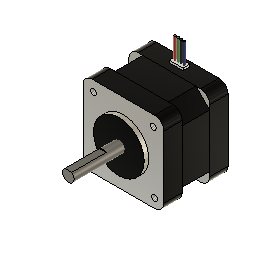
Nema14-Generic (Autodesk Fusion 360 design; units mm, degrees)
Autodesk Fusion 360 part; units mm, degrees
sketch "Profile" plane through (0, 0, 0) normal (0, 1, 0) x (1, 0, 0)
  line L0 (17.6, -17.6) -> (-17.6, -17.6)
  line L1 (-17.6, -17.6) -> (-17.6, 17.6)
  line L2 (-17.6, 17.6) -> (17.6, 17.6)
  line L3 (17.6, 17.6) -> (17.6, -17.6)
  line L4 (17.6, -17.6) -> (-17.6, 17.6) construction
  line L5 (-17.6, -17.6) -> (17.6, 17.6) construction
  circle A0 centre (0, 0) radius 11
  circle A1 centre (0, 0) radius 2.5
  line L6 (-1.5, -2) -> (1.5, -2)
  circle A2 centre (0, 0) radius 18.3848 construction
  line L7 (-11.6, -17.6) -> (-17.6, -11.6)
  line L8 (0, 0) -> (0, -17.6) construction
  line L9 (0, 0) -> (-17.6, 0) construction
  line L10 (11.6, -17.6) -> (17.6, -11.6)
  line L11 (-11.6, 17.6) -> (-17.6, 11.6)
  line L12 (11.6, 17.6) -> (17.6, 11.6)
  point P0 (0, 2.5)
  point P1 (-13, -13)
  point P2 (13, -13)
  point P3 (13, 13)
  point P4 (-13, 13)
  dimension "d1" = 35.2
  dimension "d2" = 22
  dimension "d3" = 5
  dimension "d5" = 4.5
  dimension "d8" = 26
  dimension "d18" = 6
  constraint horizontal L0
  constraint perpendicular L0 L1
  constraint parallel L0 L2
  constraint parallel L1 L3
  constraint coincident L4 A0.centre
  constraint coincident L5 A0.centre
  constraint coincident A0.centre A1.centre
  constraint equal L0 L3
  constraint coincident A1 L6.start
  constraint coincident A1 L6.end
  constraint horizontal L6
  constraint coincident A1 P0
  constraint vertical A0.centre P0
  constraint coincident A2 P1
  constraint coincident L5 P1
  constraint coincident A2 P2
  constraint coincident L4 P2
  constraint coincident A2 P3
  constraint coincident L5 P3
  constraint coincident A2 P4
  constraint coincident L4 P4
  constraint coincident L0 L7.start
  constraint coincident L1 L7.end
  constraint perpendicular L5 L7
  constraint midpoint L0 L8.end
  constraint midpoint L1 L9.end
  constraint symmetric L7.start L8 L10.start
  constraint symmetric L7.end L8 L10.end
  constraint symmetric L7.start L9 L11.start
  constraint symmetric L7.end L9 L11.end
  constraint symmetric L9 L10.start L12.start
  constraint symmetric L9 L10.end L12.end
  measures "d1" distance of L0.start L0.end
  measures "d2" diameter of A0
  measures "d3" diameter of A1
  measures "d5" distance of L6 P0
  measures "d8" distance of P1 P2
  measures "d18" distance of L0.end L7.end
extrude "Extrude1" add sketch "Profile" along normal mid plane 28 contours L0 L3 L10 | L0 L1 L2 L3 L7 L10 L11 L12 | L0 L1 L7 | L2 L3 L12 | L1 L2 L11 | A0 | A1 L6 | A1 L6 makes body 1
extrude "Extrude8" add sketch "Profile" against normal blind 2 from surface at -14 contours A0 | A1 L6 | A1 L6 bodies 1
extrude "Extrude2" add sketch "Profile" against normal blind 24 from surface at -14 separate body contours A1 L6 | A1 L6 makes body 2
extrude "Extrude3" cut sketch "Profile" along normal blind 15 from surface at -38 contours A1 L6 picked at (-0.3999, -2.0645) bodies 2 1
fillet "Fillet1" radius 4 4 edges at (-17.6, 0, 17.6) (17.6, 0, 17.6) (-17.6, 0, -17.6) (17.6, 0, -17.6) on bodies 1
extrude "Extrude5" cut sketch "Profile" along normal up to surface (-6 mm away) and the other way up to surface (-6 mm away) contours L0 L3 L10 | L0 L1 L7 | L2 L3 L12 | L1 L2 L11 bodies 1 2
ref_plane "WorkPlane1" through (14.6, 6, -14.6) normal (0, -1, 0) x (0, 0, -1)
ref_plane "WorkPlane2" through (14.6, -6, -14.6) normal (0, 1, 0) x (0, 0, 1)
split "Split1" by plane through (14.6, 6, -14.6) normal (0, -1, 0) and through (14.6, -6, -14.6) normal (0, 1, 0) bodies 1 2 makes body 3 at (17.6, -2, -3.8667) makes body 4 at (0.274, -14, 15.3897)
sketch "M3 Holes" plane through (0, -14, 0) normal (0, -1, 0) x (1, 0, 0)
  arc A0 (13.6, -17.6) -> (17.6, -13.6) centre (13.6, -13.6) ccw
  line L0 (17.6, -13.6) -> (17.6, 13.6)
  arc A1 (17.6, 13.6) -> (13.6, 17.6) centre (13.6, 13.6) ccw
  line L1 (13.6, 17.6) -> (-13.6, 17.6)
  arc A2 (-13.6, 17.6) -> (-17.6, 13.6) centre (-13.6, 13.6) ccw
  line L2 (-17.6, 13.6) -> (-17.6, -13.6)
  arc A3 (-17.6, -13.6) -> (-13.6, -17.6) centre (-13.6, -13.6) ccw
  line L3 (-13.6, -17.6) -> (13.6, -17.6)
  circle A4 centre (0, 0) radius 11
  point P0 (13, 13)
  point P1 (-13, 13)
  point P2 (-13, -13)
  point P3 (13, -13)
hole "Hole2" at (13, -14, 13) at (13.6, -14, -13.6) at (-13, -14, -13) at (-13, -14, 13) direction (0, 1, 0) diameter 2.529 depth 4 tip angle 180 bodies 4 2
thread "Thread2" "ISO Metric profile 3.0 M3x0.5 6H" major diameter 3.086 minor diameter 2.529 pitch 0.5 angle 60 resizes the face on face at (13.1259, -11.3333, 11.7418) on face at (-12.8741, -11.3333, 11.7418) on face at (-12.8741, -11.3333, -14.2582) on face at (13.7259, -11.3333, -14.8582) on bodies 4
sketch "Wire" plane through (0, 0, 17.6) normal (0, 0, 1) x (-1, 0, 0)
  line L0 (13.6, -6) -> (-13.6, -6)
  line L1 (-13.6, -6) -> (-13.6, -14)
  line L2 (-13.6, -14) -> (13.6, -14)
  line L3 (13.6, -14) -> (13.6, -6)
  line L4 (3, -12) -> (-3, -12)
  line L5 (-3, -12) -> (-3, -9)
  line L6 (-3, -9) -> (3, -9)
  line L7 (3, -9) -> (3, -12)
  circle A0 centre (2, -10.5) radius 0.5
  circle A1 centre (0.6667, -10.5) radius 0.5
  circle A2 centre (-0.6667, -10.5) radius 0.5
  circle A3 centre (-2, -10.5) radius 0.5
  line L8 (2, -10.5) -> (0.6667, -10.5) construction
  line L9 (0.6667, -10.5) -> (-0.6667, -10.5) construction
  line L10 (-0.6667, -10.5) -> (-2, -10.5) construction
  line L11 (2, -10.5) -> (3, -10.5) construction
  line L12 (-2, -10.5) -> (-3, -10.5) construction
  line L13 (0, -14) -> (0, -12) construction
  dimension "d34" = 6
  dimension "d35" = 3
  dimension "d36" = 2
  dimension "d37" = 1
  dimension "d38" = 4
  constraint horizontal L4
  constraint vertical L5
  constraint horizontal L6
  constraint vertical L7
  constraint equal A1 A2
  constraint equal A1 A3
  constraint equal A0 A3
  constraint coincident A0.centre L8.start
  constraint coincident A1.centre L8.end
  constraint horizontal L8
  constraint coincident A2.centre L9.end
  constraint parallel L8 L9
  constraint coincident A3.centre L10.end
  constraint parallel L9 L10
  constraint equal L9 L10
  constraint equal L8 L9
  constraint midpoint L7 L11.end
  constraint midpoint L5 L12.end
  constraint horizontal L12
  constraint equal L11 L12
  constraint midpoint L2 L13.start
  constraint midpoint L4 L13.end
  constraint vertical L13
  measures "d34" distance of L4.start L4.end
  measures "d35" distance of L4.end L5.end
  measures "d36" distance of L13.start L13.end
  measures "d37" diameter of A0
  measures "d38" distance of A0.centre A3.centre
extrude "Extrude6" add sketch "Wire" along normal blind 1 separate body contours L4 L5 L6 L7 | A0 | A1 | A2 | A3 makes body 5
extrude "Extrude7" add sketch "Wire" along normal blind 10 separate body contours A0 | A1 | A2 | A3 makes body 6 at (-1.166, 10.5249, 24.2667) makes body 7 at (0.1673, 10.5249, 24.2667) makes body 8 at (-2.4994, 10.5249, 24.2667) makes body 9 at (1.5006, 10.5249, 24.2667)
equation "MotorLength = 28 mm"
named bodies: "Rear Cap", "Center Section", "Front Cap", "Wire Grommet", "A2", "B1", "A1", "B2", "Shaft"
